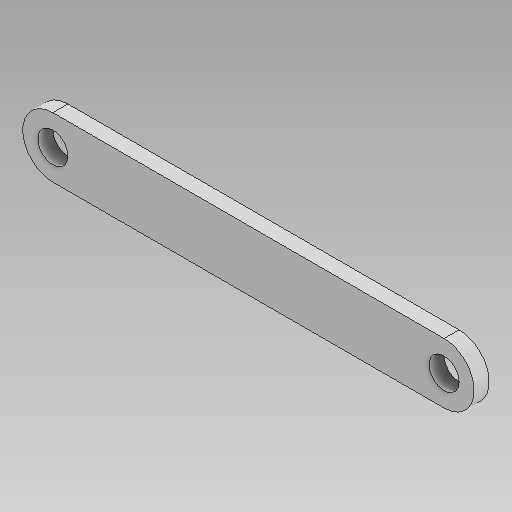
# Autodesk Inventor part: link_l1
Saved by Autodesk Inventor 2025 (Build 290162000, 162)
## iProperties
Created: 2024-09-22
Part Number: link_l1
Material: 일반
Document SubType Name: Modeling
Designer: OSB
Density: 1 g/cm^3
Appearance: 기본값
Author: OSB
Autodesk Inventor part; units mm, degrees
ref_plane "YZ Plane" through (0, 0, 0) normal (1, 0, 0) x (0, 1, 0)
ref_plane "XZ Plane" through (0, 0, 0) normal (0, 1, 0) x (-1, 0, 0)
ref_plane "XY Plane" through (0, 0, 0) normal (0, 0, 1) x (1, 0, 0)
sketch "스케치1" plane through (0, 0, 0) normal (0, 0, 1) x (1, 0, 0)
  line L0 (-65, 0) -> (65, 0) construction
  line L1 (-65, -10) -> (65, -10)
  line L2 (65, 10) -> (-65, 10)
  arc A0 (-65, 10) -> (-65, -10) centre (-65, 0) ccw
  arc A1 (65, -10) -> (65, 10) centre (65, 0) ccw
  circle A2 centre (-65, 0) radius 5
  circle A3 centre (65, 0) radius 5
  point P0 (0, 0)
  dimension "d1" = 20
  dimension "d2" = 10
  dimension "d3" = 10
  dimension "d4" = 130
  constraints: 8 end point, 4 centre point, 4 point on circle, 4 tangent, 2 coincident, 1 horizontal, 1 midpoint, 1 parallel
  measures "d1" diameter of A1
  measures "d2" diameter of A2
  measures "d3" diameter of A3
  measures "d4" distance of L0.end L0.start
extrude "돌출1" add sketch "스케치1" along normal blind 5
